New Bottom Plate_v3 (Autodesk Fusion 360 design; units mm, degrees)
Autodesk Fusion 360 part; units mm, degrees
note: some values were not read from the file. Set by a fixed rule: which sketch regions a step uses.
sketch "Reference" plane through (0, 0, 0) normal (0, 0, 1) x (1, 0, 0)
  line L0 (298.2751, -95.25) -> (298.2751, -113.3)
  line L1 (298.275, 1) -> (298.275, -57.15)
  line L2 (298.275, -57.15) -> (298.275, -57.15)
  line L3 (304.5217, -115.3) -> (303.775, 3)
  line L4 (179.47, 0) -> (290.235, 0)
  line L5 (290.2351, -112.3) -> (230.642, -112.3)
  line L6 (290.235, 1) -> (298.275, 1)
  line L7 (290.235, 0) -> (298.275, 0)
  line L8 (290.2351, -112.3) -> (298.2751, -112.3)
  arc A0 (302.0217, -117.8) -> (304.5217, -115.3) centre (302.0374, -115.3157) ccw
  line L9 (298.2751, -57.15) -> (298.2751, -74.2)
  line L10 (171.43, 0) -> (171.43, 1)
  line L11 (230.642, -112.3) -> (230.642, -113.3)
  line L12 (222.602, -113.3) -> (222.602, -112.3)
  arc A1 (303.775, 3) -> (301.275, 5.5) centre (301.275, 3) ccw
  line L13 (-28.337, -112.3) -> (-29.3375, -112.3)
  line L14 (-28.3375, 1.5) -> (-28.3375, 3)
  line L15 (-28.337, 1.5) -> (-6.3413, 1.5)
  line L16 (230.642, -112.3) -> (230.642, -113.3)
  line L17 (230.642, -113.3) -> (222.602, -113.3)
  line L18 (-36.12, -117.7958) -> (-31.338, -117.8)
  line L19 (222.602, -113.3) -> (222.602, -112.3)
  line L20 (-28.337, -113.3) -> (-28.337, -112.3)
  line L21 (-29.3375, -113.3) -> (-29.338, -113.3)
  arc A2 (-38.6178, -115.2937) -> (-36.12, -117.7958) centre (-36.1178, -115.2958) ccw
  line L22 (57.336, -112.3) -> (-20.297, -112.3)
  line L23 (8.02, 1) -> (8.02, 0)
  line L24 (-29.3375, -112.3) -> (-29.3375, -113.3)
  line L25 (-33.0995, -112.3) -> (-33.0995, 1.5)
  line L26 (-29.338, -112.3) -> (-33.0995, -112.3)
  line L27 (57.336, -113.3) -> (57.336, -112.3)
  line L28 (-20.297, -113.3) -> (-28.337, -113.3)
  line L29 (-29.338, -113.3) -> (-29.338, -112.3)
  line L30 (-20.297, -112.3) -> (-20.297, -113.3)
  line L31 (301.275, 5.5) -> (-36.0995, 5.5)
  line L32 (-38.5995, -94.25) -> (-38.6178, -115.2937)
  line L33 (298.2751, -76.2) -> (298.2751, -93.25)
  line L34 (298.275, -95.25) -> (298.275, -95.25)
  line L35 (298.275, -76.2) -> (298.275, -76.2)
  line L36 (-6.3413, 1.5) -> (-6.3413, 0)
  line L37 (-38.5995, 3) -> (-38.5995, -94.25)
  arc A3 (303.775, 3) -> (301.275, 5.5) centre (301.275, 3) ccw
  line L38 (298.2751, -74.2) -> (298.275, -74.2)
  line L39 (-28.337, 3) -> (-28.337, 1.5)
  line L40 (-33.0995, 1.5) -> (-28.3375, 1.5)
  line L41 (-0.02, 0) -> (-0.02, 1)
  arc A4 (-36.0995, 5.5) -> (-38.5995, 3) centre (-36.0995, 3) ccw
  line L42 (-31.338, -117.8) -> (302.0217, -117.8)
  line L43 (-6.3413, 0) -> (-0.02, 0)
  line L44 (298.275, -57.15) -> (298.275, -57.15)
  line L45 (-0.02, 1) -> (8.02, 1)
  line L46 (8.02, 0) -> (171.43, 0)
  line L47 (-28.3375, 3) -> (-28.337, 3)
  line L48 (290.235, 0) -> (290.235, 1)
  line L49 (290.235, 1) -> (298.275, 1)
  line L50 (298.2751, -57.15) -> (298.2751, -74.2)
  line L51 (298.275, 1) -> (298.275, -57.15)
  line L52 (222.602, -112.3) -> (65.376, -112.3)
  line L53 (-33.0995, -112.3) -> (-33.0995, 1.5)
  line L54 (301.275, 5.5) -> (-36.0995, 5.5)
  line L55 (-31.338, -117.8) -> (302.0217, -117.8)
  line L56 (57.336, -112.3) -> (-20.297, -112.3)
  line L57 (8.02, 0) -> (171.43, 0)
  line L58 (290.2351, -112.3) -> (230.642, -112.3)
  line L59 (298.2751, -95.25) -> (298.2751, -113.3)
  line L60 (298.275, -76.2) -> (298.275, -76.2)
  line L61 (298.275, -74.2) -> (298.275, -76.2)
  line L62 (298.2751, -76.2) -> (298.2751, -93.25)
  line L63 (298.2751, -93.25) -> (298.275, -93.25)
  line L64 (298.275, -93.25) -> (298.275, -95.25)
  line L65 (290.2351, -113.3) -> (290.2351, -112.3)
  arc A5 (302.0217, -117.8) -> (304.5217, -115.3) centre (302.0374, -115.3157) ccw
  line L66 (179.47, 0) -> (290.235, 0)
  line L67 (298.2751, -113.3) -> (290.2351, -113.3)
  line L68 (304.5217, -115.3) -> (303.775, 3)
  line L69 (298.275, -95.25) -> (298.275, -95.25)
  line L70 (57.336, -113.3) -> (57.336, -112.3)
  line L71 (65.376, -113.3) -> (57.336, -113.3)
  line L72 (-29.338, -113.3) -> (-29.338, -112.3)
  line L73 (-6.3413, 1.5) -> (-6.3413, 0)
  line L74 (-29.3375, -113.3) -> (-29.338, -113.3)
  line L75 (-29.3375, -112.3) -> (-29.3375, -113.3)
  line L76 (-28.3375, 1.5) -> (-28.3375, 3)
  line L77 (-28.337, 1.5) -> (-6.3413, 1.5)
  line L78 (-28.337, -112.3) -> (-29.3375, -112.3)
  line L79 (-28.337, -113.3) -> (-28.337, -112.3)
  line L80 (-28.3375, 3) -> (-28.337, 3)
  line L81 (-20.297, -113.3) -> (-28.337, -113.3)
  line L82 (65.376, -112.3) -> (65.376, -113.3)
  line L83 (-20.297, -112.3) -> (-20.297, -113.3)
  line L84 (-29.338, -112.3) -> (-33.0995, -112.3)
  line L85 (8.02, 1) -> (8.02, 0)
  line L86 (-28.337, 3) -> (-28.337, 1.5)
  arc A6 (-38.6178, -115.2937) -> (-36.12, -117.7958) centre (-36.1178, -115.2958) ccw
  line L87 (-38.5995, -94.25) -> (-38.6178, -115.2937)
  line L88 (-38.5995, 3) -> (-38.5995, -94.25)
  line L89 (-0.02, 0) -> (-0.02, 1)
  line L90 (-33.0995, 1.5) -> (-28.3375, 1.5)
  line L91 (-6.3413, 0) -> (-0.02, 0)
  arc A7 (-36.0995, 5.5) -> (-38.5995, 3) centre (-36.0995, 3) ccw
  line L92 (-0.02, 1) -> (8.02, 1)
  line L93 (-36.12, -117.7958) -> (-31.338, -117.8)
  line L94 (298.275, -93.25) -> (298.275, -95.25)
  line L95 (298.2751, -113.3) -> (290.2351, -113.3)
  line L96 (290.2351, -113.3) -> (290.2351, -112.3)
  line L97 (298.2751, -93.25) -> (298.275, -93.25)
  line L98 (298.275, -74.2) -> (298.275, -76.2)
  line L99 (298.2751, -74.2) -> (298.275, -74.2)
  line L100 (290.235, 0) -> (290.235, 1)
  line L101 (179.47, 1) -> (179.47, 0)
  line L102 (230.642, -113.3) -> (222.602, -113.3)
  line L103 (179.47, 1) -> (179.47, 0)
  line L104 (171.43, 1) -> (179.47, 1)
  line L105 (222.602, -112.3) -> (65.376, -112.3)
  line L106 (65.376, -112.3) -> (65.376, -113.3)
  line L107 (65.376, -113.3) -> (57.336, -113.3)
  line L108 (171.43, 0) -> (171.43, 1)
  line L109 (171.43, 1) -> (179.47, 1)
  dimension "d29" = 5.5
  dimension "d30" = 5.5
  dimension "d31" = 6.2339
  dimension "d32" = 5.5125
  dimension "d33" = 5.5
  dimension "d34" = 6.2276
  dimension "d35" = 5.5188
  constraint coincident L5.start L8.start
  constraint perpendicular L0 L8
  constraint coincident L8.end L59
  constraint coincident L4.end L7.start
  constraint perpendicular L7 L48
  constraint coincident L7.end L51
  measures "d29" distance of L42 L58
  measures "d30" distance of L4 L31
  measures "d31" distance of L0.end L3
  measures "d32" distance of L1.start L3
  measures "d33" distance of L25 L37
  measures "d34" distance of L8.end L3
  measures "d35" distance of L7.end L68
sketch "FlatPlateSketch" plane through (0, 0, 0) normal (0, 0, 1) x (1, 0, 0)
  line L0 (298.2751, -95.25) -> (298.2751, -113.3)
  line L1 (298.275, 1) -> (298.275, -57.15)
  line L2 (298.275, -57.15) -> (298.275, -57.15)
  line L3 (304.5217, -115.3) -> (303.775, 3)
  line L4 (179.47, 0) -> (290.235, 0)
  line L5 (290.2351, -112.3) -> (230.642, -112.3)
  line L6 (290.235, 1) -> (298.275, 1)
  line L7 (290.235, 0) -> (298.275, 0)
  line L8 (290.2351, -112.3) -> (298.2751, -112.3)
  arc A0 (302.0217, -117.8) -> (304.5217, -115.3) centre (302.0374, -115.3157) ccw
  line L9 (298.2751, -57.15) -> (298.2751, -74.2)
  line L10 (171.43, 0) -> (171.43, 1)
  line L11 (230.642, -112.3) -> (230.642, -113.3)
  line L12 (222.602, -113.3) -> (222.602, -112.3)
  arc A1 (303.775, 3) -> (301.275, 5.5) centre (301.275, 3) ccw
  line L13 (-28.337, -112.3) -> (-29.3375, -112.3)
  line L14 (-28.3375, 1.5) -> (-28.3375, 3)
  line L15 (-28.337, 1.5) -> (-6.3413, 1.5)
  line L16 (230.642, -112.3) -> (230.642, -113.3)
  line L17 (230.642, -113.3) -> (222.602, -113.3)
  line L18 (-36.12, -117.7958) -> (-31.338, -117.8)
  line L19 (222.602, -113.3) -> (222.602, -112.3)
  line L20 (-28.337, -113.3) -> (-28.337, -112.3)
  line L21 (-29.3375, -113.3) -> (-29.338, -113.3)
  arc A2 (-38.6178, -115.2937) -> (-36.12, -117.7958) centre (-36.1178, -115.2958) ccw
  line L22 (57.336, -112.3) -> (-20.297, -112.3)
  line L23 (8.02, 1) -> (8.02, 0)
  line L24 (-29.3375, -112.3) -> (-29.3375, -113.3)
  line L25 (-33.0995, -112.3) -> (-33.0995, 1.5)
  line L26 (-29.338, -112.3) -> (-33.0995, -112.3)
  line L27 (57.336, -113.3) -> (57.336, -112.3)
  line L28 (-20.297, -113.3) -> (-28.337, -113.3)
  line L29 (-29.338, -113.3) -> (-29.338, -112.3)
  line L30 (-20.297, -112.3) -> (-20.297, -113.3)
  line L31 (301.275, 5.5) -> (-36.0995, 5.5)
  line L32 (-38.5995, -94.25) -> (-38.6178, -115.2937)
  line L33 (298.2751, -76.2) -> (298.2751, -93.25)
  line L34 (298.275, -95.25) -> (298.275, -95.25)
  line L35 (298.275, -76.2) -> (298.275, -76.2)
  line L36 (-6.3413, 1.5) -> (-6.3413, 0)
  line L37 (-38.5995, 3) -> (-38.5995, -94.25)
  arc A3 (303.775, 3) -> (301.275, 5.5) centre (301.275, 3) ccw
  line L38 (298.2751, -74.2) -> (298.275, -74.2)
  line L39 (-28.337, 3) -> (-28.337, 1.5)
  line L40 (-33.0995, 1.5) -> (-28.3375, 1.5)
  line L41 (-0.02, 0) -> (-0.02, 1)
  arc A4 (-36.0995, 5.5) -> (-38.5995, 3) centre (-36.0995, 3) ccw
  line L42 (-31.338, -117.8) -> (302.0217, -117.8)
  line L43 (-6.3413, 0) -> (-0.02, 0)
  line L44 (298.275, -57.15) -> (298.275, -57.15)
  line L45 (-0.02, 1) -> (8.02, 1)
  line L46 (8.02, 0) -> (171.43, 0)
  line L47 (-28.3375, 3) -> (-28.337, 3)
  line L48 (290.235, 0) -> (290.235, 1)
  line L49 (290.235, 1) -> (298.275, 1)
  line L50 (298.2751, -57.15) -> (298.2751, -74.2)
  line L51 (298.275, 1) -> (298.275, -57.15)
  line L52 (222.602, -112.3) -> (65.376, -112.3)
  line L53 (-33.0995, -112.3) -> (-33.0995, 1.5)
  line L54 (301.275, 5.5) -> (-36.0995, 5.5)
  line L55 (-31.338, -117.8) -> (302.0217, -117.8)
  line L56 (57.336, -112.3) -> (-20.297, -112.3)
  line L57 (8.02, 0) -> (171.43, 0)
  line L58 (290.2351, -112.3) -> (230.642, -112.3)
  line L59 (298.2751, -95.25) -> (298.2751, -113.3)
  line L60 (298.275, -76.2) -> (298.275, -76.2)
  line L61 (298.275, -74.2) -> (298.275, -76.2)
  line L62 (298.2751, -76.2) -> (298.2751, -93.25)
  line L63 (298.2751, -93.25) -> (298.275, -93.25)
  line L64 (298.275, -93.25) -> (298.275, -95.25)
  line L65 (290.2351, -113.3) -> (290.2351, -112.3)
  arc A5 (302.0217, -117.8) -> (304.5217, -115.3) centre (302.0374, -115.3157) ccw
  line L66 (179.47, 0) -> (290.235, 0)
  line L67 (298.2751, -113.3) -> (290.2351, -113.3)
  line L68 (304.5217, -115.3) -> (303.775, 3)
  line L69 (298.275, -95.25) -> (298.275, -95.25)
  line L70 (57.336, -113.3) -> (57.336, -112.3)
  line L71 (65.376, -113.3) -> (57.336, -113.3)
  line L72 (-29.338, -113.3) -> (-29.338, -112.3)
  line L73 (-6.3413, 1.5) -> (-6.3413, 0)
  line L74 (-29.3375, -113.3) -> (-29.338, -113.3)
  line L75 (-29.3375, -112.3) -> (-29.3375, -113.3)
  line L76 (-28.3375, 1.5) -> (-28.3375, 3)
  line L77 (-28.337, 1.5) -> (-6.3413, 1.5)
  line L78 (-28.337, -112.3) -> (-29.3375, -112.3)
  line L79 (-28.337, -113.3) -> (-28.337, -112.3)
  line L80 (-28.3375, 3) -> (-28.337, 3)
  line L81 (-20.297, -113.3) -> (-28.337, -113.3)
  line L82 (65.376, -112.3) -> (65.376, -113.3)
  line L83 (-20.297, -112.3) -> (-20.297, -113.3)
  line L84 (-29.338, -112.3) -> (-33.0995, -112.3)
  line L85 (8.02, 1) -> (8.02, 0)
  line L86 (-28.337, 3) -> (-28.337, 1.5)
  arc A6 (-38.6178, -115.2937) -> (-36.12, -117.7958) centre (-36.1178, -115.2958) ccw
  line L87 (-38.5995, -94.25) -> (-38.6178, -115.2937)
  line L88 (-38.5995, 3) -> (-38.5995, -94.25)
  line L89 (-0.02, 0) -> (-0.02, 1)
  line L90 (-33.0995, 1.5) -> (-28.3375, 1.5)
  line L91 (-6.3413, 0) -> (-0.02, 0)
  arc A7 (-36.0995, 5.5) -> (-38.5995, 3) centre (-36.0995, 3) ccw
  line L92 (-0.02, 1) -> (8.02, 1)
  line L93 (-36.12, -117.7958) -> (-31.338, -117.8)
  line L94 (298.275, -93.25) -> (298.275, -95.25)
  line L95 (298.2751, -113.3) -> (290.2351, -113.3)
  line L96 (290.2351, -113.3) -> (290.2351, -112.3)
  line L97 (298.2751, -93.25) -> (298.275, -93.25)
  line L98 (298.275, -74.2) -> (298.275, -76.2)
  line L99 (298.2751, -74.2) -> (298.275, -74.2)
  line L100 (290.235, 0) -> (290.235, 1)
  line L101 (179.47, 1) -> (179.47, 0)
  line L102 (230.642, -113.3) -> (222.602, -113.3)
  line L103 (179.47, 1) -> (179.47, 0)
  line L104 (171.43, 1) -> (179.47, 1)
  line L105 (222.602, -112.3) -> (65.376, -112.3)
  line L106 (65.376, -112.3) -> (65.376, -113.3)
  line L107 (65.376, -113.3) -> (57.336, -113.3)
  line L108 (171.43, 0) -> (171.43, 1)
  line L109 (171.43, 1) -> (179.47, 1)
  dimension "d36" = 5.5
  dimension "d37" = 5.5
  dimension "d38" = 6.2339
  dimension "d39" = 5.5125
  dimension "d40" = 5.5
  dimension "d41" = 6.2276
  dimension "d42" = 5.5188
  constraint coincident L5.start L8.start
  constraint perpendicular L0 L8
  constraint coincident L8.end L59
  constraint coincident L4.end L7.start
  constraint perpendicular L7 L48
  constraint coincident L7.end L51
  measures "d36" distance of L42 L58
  measures "d37" distance of L4 L31
  measures "d38" distance of L0.end L3
  measures "d39" distance of L1.start L3
  measures "d40" distance of L25 L37
  measures "d41" distance of L8.end L3
  measures "d42" distance of L7.end L68
sketch "Sketch7" plane through (0, 0, 0) normal (0, 0, 1) x (1, 0, 0)
  line L0 (298.2751, -95.25) -> (298.2751, -113.3)
  line L1 (298.275, 1) -> (298.275, -57.15)
  line L2 (298.275, -57.15) -> (298.275, -57.15)
  line L3 (304.5217, -115.3) -> (303.775, 3)
  line L4 (179.47, 0) -> (290.235, 0)
  line L5 (290.2351, -112.3) -> (230.642, -112.3)
  line L6 (290.235, 1) -> (298.275, 1)
  line L7 (290.235, 0) -> (298.275, 0)
  line L8 (290.2351, -112.3) -> (298.2751, -112.3)
  arc A0 (302.0217, -117.8) -> (304.5217, -115.3) centre (302.0374, -115.3157) ccw
  line L9 (298.2751, -57.15) -> (298.2751, -74.2)
  line L10 (171.43, 0) -> (171.43, 1)
  line L11 (230.642, -112.3) -> (230.642, -113.3)
  line L12 (222.602, -113.3) -> (222.602, -112.3)
  arc A1 (303.775, 3) -> (301.275, 5.5) centre (301.275, 3) ccw
  line L13 (-28.337, -112.3) -> (-29.3375, -112.3)
  line L14 (-28.3375, 1.5) -> (-28.3375, 3)
  line L15 (-28.337, 1.5) -> (-6.3413, 1.5)
  line L16 (230.642, -112.3) -> (230.642, -113.3)
  line L17 (230.642, -113.3) -> (222.602, -113.3)
  line L18 (-36.12, -117.7958) -> (-31.338, -117.8)
  line L19 (222.602, -113.3) -> (222.602, -112.3)
  line L20 (-28.337, -113.3) -> (-28.337, -112.3)
  line L21 (-29.3375, -113.3) -> (-29.338, -113.3)
  arc A2 (-38.6178, -115.2937) -> (-36.12, -117.7958) centre (-36.1178, -115.2958) ccw
  line L22 (57.336, -112.3) -> (-20.297, -112.3)
  line L23 (8.02, 1) -> (8.02, 0)
  line L24 (-29.3375, -112.3) -> (-29.3375, -113.3)
  line L25 (-33.0995, -112.3) -> (-33.0995, 1.5)
  line L26 (-29.338, -112.3) -> (-33.0995, -112.3)
  line L27 (57.336, -113.3) -> (57.336, -112.3)
  line L28 (-20.297, -113.3) -> (-28.337, -113.3)
  line L29 (-29.338, -113.3) -> (-29.338, -112.3)
  line L30 (-20.297, -112.3) -> (-20.297, -113.3)
  line L31 (301.275, 5.5) -> (-36.0995, 5.5)
  line L32 (-38.5995, -94.25) -> (-38.6178, -115.2937)
  line L33 (298.2751, -76.2) -> (298.2751, -93.25)
  line L34 (298.275, -95.25) -> (298.275, -95.25)
  line L35 (298.275, -76.2) -> (298.275, -76.2)
  line L36 (-6.3413, 1.5) -> (-6.3413, 0)
  line L37 (-38.5995, 3) -> (-38.5995, -94.25)
  arc A3 (303.775, 3) -> (301.275, 5.5) centre (301.275, 3) ccw
  line L38 (298.2751, -74.2) -> (298.275, -74.2)
  line L39 (-28.337, 3) -> (-28.337, 1.5)
  line L40 (-33.0995, 1.5) -> (-28.3375, 1.5)
  line L41 (-0.02, 0) -> (-0.02, 1)
  arc A4 (-36.0995, 5.5) -> (-38.5995, 3) centre (-36.0995, 3) ccw
  line L42 (-31.338, -117.8) -> (302.0217, -117.8)
  line L43 (-6.3413, 0) -> (-0.02, 0)
  line L44 (298.275, -57.15) -> (298.275, -57.15)
  line L45 (-0.02, 1) -> (8.02, 1)
  line L46 (8.02, 0) -> (171.43, 0)
  line L47 (-28.3375, 3) -> (-28.337, 3)
  line L48 (290.235, 0) -> (290.235, 1)
  line L49 (290.235, 1) -> (298.275, 1)
  line L50 (298.2751, -57.15) -> (298.2751, -74.2)
  line L51 (298.275, 1) -> (298.275, -57.15)
  line L52 (222.602, -112.3) -> (65.376, -112.3)
  line L53 (-33.0995, -112.3) -> (-33.0995, 1.5)
  line L54 (301.275, 5.5) -> (-36.0995, 5.5)
  line L55 (-31.338, -117.8) -> (302.0217, -117.8)
  line L56 (57.336, -112.3) -> (-20.297, -112.3)
  line L57 (8.02, 0) -> (171.43, 0)
  line L58 (290.2351, -112.3) -> (230.642, -112.3)
  line L59 (298.2751, -95.25) -> (298.2751, -113.3)
  line L60 (298.275, -76.2) -> (298.275, -76.2)
  line L61 (298.275, -74.2) -> (298.275, -76.2)
  line L62 (298.2751, -76.2) -> (298.2751, -93.25)
  line L63 (298.2751, -93.25) -> (298.275, -93.25)
  line L64 (298.275, -93.25) -> (298.275, -95.25)
  line L65 (290.2351, -113.3) -> (290.2351, -112.3)
  arc A5 (302.0217, -117.8) -> (304.5217, -115.3) centre (302.0374, -115.3157) ccw
  line L66 (179.47, 0) -> (290.235, 0)
  line L67 (298.2751, -113.3) -> (290.2351, -113.3)
  line L68 (304.5217, -115.3) -> (303.775, 3)
  line L69 (298.275, -95.25) -> (298.275, -95.25)
  line L70 (57.336, -113.3) -> (57.336, -112.3)
  line L71 (65.376, -113.3) -> (57.336, -113.3)
  line L72 (-29.338, -113.3) -> (-29.338, -112.3)
  line L73 (-6.3413, 1.5) -> (-6.3413, 0)
  line L74 (-29.3375, -113.3) -> (-29.338, -113.3)
  line L75 (-29.3375, -112.3) -> (-29.3375, -113.3)
  line L76 (-28.3375, 1.5) -> (-28.3375, 3)
  line L77 (-28.337, 1.5) -> (-6.3413, 1.5)
  line L78 (-28.337, -112.3) -> (-29.3375, -112.3)
  line L79 (-28.337, -113.3) -> (-28.337, -112.3)
  line L80 (-28.3375, 3) -> (-28.337, 3)
  line L81 (-20.297, -113.3) -> (-28.337, -113.3)
  line L82 (65.376, -112.3) -> (65.376, -113.3)
  line L83 (-20.297, -112.3) -> (-20.297, -113.3)
  line L84 (-29.338, -112.3) -> (-33.0995, -112.3)
  line L85 (8.02, 1) -> (8.02, 0)
  line L86 (-28.337, 3) -> (-28.337, 1.5)
  arc A6 (-38.6178, -115.2937) -> (-36.12, -117.7958) centre (-36.1178, -115.2958) ccw
  line L87 (-38.5995, -94.25) -> (-38.6178, -115.2937)
  line L88 (-38.5995, 3) -> (-38.5995, -94.25)
  line L89 (-0.02, 0) -> (-0.02, 1)
  line L90 (-33.0995, 1.5) -> (-28.3375, 1.5)
  line L91 (-6.3413, 0) -> (-0.02, 0)
  arc A7 (-36.0995, 5.5) -> (-38.5995, 3) centre (-36.0995, 3) ccw
  line L92 (-0.02, 1) -> (8.02, 1)
  line L93 (-36.12, -117.7958) -> (-31.338, -117.8)
  line L94 (298.275, -93.25) -> (298.275, -95.25)
  line L95 (298.2751, -113.3) -> (290.2351, -113.3)
  line L96 (290.2351, -113.3) -> (290.2351, -112.3)
  line L97 (298.2751, -93.25) -> (298.275, -93.25)
  line L98 (298.275, -74.2) -> (298.275, -76.2)
  line L99 (298.2751, -74.2) -> (298.275, -74.2)
  line L100 (290.235, 0) -> (290.235, 1)
  line L101 (179.47, 1) -> (179.47, 0)
  line L102 (230.642, -113.3) -> (222.602, -113.3)
  line L103 (179.47, 1) -> (179.47, 0)
  line L104 (171.43, 1) -> (179.47, 1)
  line L105 (222.602, -112.3) -> (65.376, -112.3)
  line L106 (65.376, -112.3) -> (65.376, -113.3)
  line L107 (65.376, -113.3) -> (57.336, -113.3)
  line L108 (171.43, 0) -> (171.43, 1)
  line L109 (171.43, 1) -> (179.47, 1)
  dimension "d45" = 5.5
  dimension "d46" = 5.5
  dimension "d47" = 6.2339
  dimension "d48" = 5.5125
  dimension "d49" = 5.5
  dimension "d50" = 6.2276
  dimension "d51" = 5.5188
  constraint coincident L5.start L8.start
  constraint perpendicular L0 L8
  constraint coincident L8.end L59
  constraint coincident L4.end L7.start
  constraint perpendicular L7 L48
  constraint coincident L7.end L51
  measures "d45" distance of L42 L58
  measures "d46" distance of L4 L31
  measures "d47" distance of L0.end L3
  measures "d48" distance of L1.start L3
  measures "d49" distance of L25 L37
  measures "d50" distance of L8.end L3
  measures "d51" distance of L7.end L68
extrude "Extrude4" add sketch "FlatPlateSketch" against normal blind 1 contours L0 L1 L4 L5 L7 L8 L9 L10 L11 L12 L13 L15 L16 L17 L19 L20 L22 L23 L25 L26 L27 L28 L30 L33 L36 L40 L41 L43 L45 L46 L50 L51 L52 L53 L56 L57 L58 L59 L61 L62 L64 L66 L70 L71 L73 L77 L78 L79 L81 L82 L83 L84 L85 L89 L90 L91 L92 L94 L98 L101 L102 L103 L104 L105 L106 L107 L108 L109 | L0 L8 L59 L65 L67 L95 L96 | L1 L6 L7 L48 L49 L51 L100 | L3 A0 A1 L18 A2 L31 L32 L37 A3 A4 L42 L54 L55 A5 L68 A6 L87 L88 A7 L93
sketch "Sketch8" plane through (0, 0, 0) normal (0, 0, 1) x (1, 0, 0)
  line L0 (298.2751, -95.25) -> (298.2751, -113.3)
  line L1 (298.275, 1) -> (298.275, -57.15)
  line L2 (298.275, -57.15) -> (298.275, -57.15)
  line L3 (304.5217, -115.3) -> (303.775, 3)
  line L4 (179.47, 0) -> (290.235, 0)
  line L5 (290.2351, -112.3) -> (230.642, -112.3)
  line L6 (290.235, 1) -> (298.275, 1)
  line L7 (290.235, 0) -> (298.275, 0)
  line L8 (290.2351, -112.3) -> (298.2751, -112.3)
  arc A0 (302.0217, -117.8) -> (304.5217, -115.3) centre (302.0374, -115.3157) ccw
  line L9 (298.2751, -57.15) -> (298.2751, -74.2)
  line L10 (171.43, 0) -> (171.43, 1)
  line L11 (230.642, -112.3) -> (230.642, -113.3)
  line L12 (222.602, -113.3) -> (222.602, -112.3)
  arc A1 (303.775, 3) -> (301.275, 5.5) centre (301.275, 3) ccw
  line L13 (-28.337, -112.3) -> (-29.3375, -112.3)
  line L14 (-28.3375, 1.5) -> (-28.3375, 3)
  line L15 (-28.337, 1.5) -> (-6.3413, 1.5)
  line L16 (230.642, -112.3) -> (230.642, -113.3)
  line L17 (230.642, -113.3) -> (222.602, -113.3)
  line L18 (-36.12, -117.7958) -> (-31.338, -117.8)
  line L19 (222.602, -113.3) -> (222.602, -112.3)
  line L20 (-28.337, -113.3) -> (-28.337, -112.3)
  line L21 (-29.3375, -113.3) -> (-29.338, -113.3)
  arc A2 (-38.6178, -115.2937) -> (-36.12, -117.7958) centre (-36.1178, -115.2958) ccw
  line L22 (57.336, -112.3) -> (-20.297, -112.3)
  line L23 (8.02, 1) -> (8.02, 0)
  line L24 (-29.3375, -112.3) -> (-29.3375, -113.3)
  line L25 (-33.0995, -112.3) -> (-33.0995, 1.5)
  line L26 (-29.338, -112.3) -> (-33.0995, -112.3)
  line L27 (57.336, -113.3) -> (57.336, -112.3)
  line L28 (-20.297, -113.3) -> (-28.337, -113.3)
  line L29 (-29.338, -113.3) -> (-29.338, -112.3)
  line L30 (-20.297, -112.3) -> (-20.297, -113.3)
  line L31 (301.275, 5.5) -> (-36.0995, 5.5)
  line L32 (-38.5995, -94.25) -> (-38.6178, -115.2937)
  line L33 (298.2751, -76.2) -> (298.2751, -93.25)
  line L34 (298.275, -95.25) -> (298.275, -95.25)
  line L35 (298.275, -76.2) -> (298.275, -76.2)
  line L36 (-6.3413, 1.5) -> (-6.3413, 0)
  line L37 (-38.5995, 3) -> (-38.5995, -94.25)
  arc A3 (303.775, 3) -> (301.275, 5.5) centre (301.275, 3) ccw
  line L38 (298.2751, -74.2) -> (298.275, -74.2)
  line L39 (-28.337, 3) -> (-28.337, 1.5)
  line L40 (-33.0995, 1.5) -> (-28.3375, 1.5)
  line L41 (-0.02, 0) -> (-0.02, 1)
  arc A4 (-36.0995, 5.5) -> (-38.5995, 3) centre (-36.0995, 3) ccw
  line L42 (-31.338, -117.8) -> (302.0217, -117.8)
  line L43 (-6.3413, 0) -> (-0.02, 0)
  line L44 (298.275, -57.15) -> (298.275, -57.15)
  line L45 (-0.02, 1) -> (8.02, 1)
  line L46 (8.02, 0) -> (171.43, 0)
  line L47 (-28.3375, 3) -> (-28.337, 3)
  line L48 (290.235, 0) -> (290.235, 1)
  line L49 (290.235, 1) -> (298.275, 1)
  line L50 (298.2751, -57.15) -> (298.2751, -74.2)
  line L51 (298.275, 1) -> (298.275, -57.15)
  line L52 (222.602, -112.3) -> (65.376, -112.3)
  line L53 (-33.0995, -112.3) -> (-33.0995, 1.5)
  line L54 (301.275, 5.5) -> (-36.0995, 5.5)
  line L55 (-31.338, -117.8) -> (302.0217, -117.8)
  line L56 (57.336, -112.3) -> (-20.297, -112.3)
  line L57 (8.02, 0) -> (171.43, 0)
  line L58 (290.2351, -112.3) -> (230.642, -112.3)
  line L59 (298.2751, -95.25) -> (298.2751, -113.3)
  line L60 (298.275, -76.2) -> (298.275, -76.2)
  line L61 (298.275, -74.2) -> (298.275, -76.2)
  line L62 (298.2751, -76.2) -> (298.2751, -93.25)
  line L63 (298.2751, -93.25) -> (298.275, -93.25)
  line L64 (298.275, -93.25) -> (298.275, -95.25)
  line L65 (290.2351, -113.3) -> (290.2351, -112.3)
  arc A5 (302.0217, -117.8) -> (304.5217, -115.3) centre (302.0374, -115.3157) ccw
  line L66 (179.47, 0) -> (290.235, 0)
  line L67 (298.2751, -113.3) -> (290.2351, -113.3)
  line L68 (304.5217, -115.3) -> (303.775, 3)
  line L69 (298.275, -95.25) -> (298.275, -95.25)
  line L70 (57.336, -113.3) -> (57.336, -112.3)
  line L71 (65.376, -113.3) -> (57.336, -113.3)
  line L72 (-29.338, -113.3) -> (-29.338, -112.3)
  line L73 (-6.3413, 1.5) -> (-6.3413, 0)
  line L74 (-29.3375, -113.3) -> (-29.338, -113.3)
  line L75 (-29.3375, -112.3) -> (-29.3375, -113.3)
  line L76 (-28.3375, 1.5) -> (-28.3375, 3)
  line L77 (-28.337, 1.5) -> (-6.3413, 1.5)
  line L78 (-28.337, -112.3) -> (-29.3375, -112.3)
  line L79 (-28.337, -113.3) -> (-28.337, -112.3)
  line L80 (-28.3375, 3) -> (-28.337, 3)
  line L81 (-20.297, -113.3) -> (-28.337, -113.3)
  line L82 (65.376, -112.3) -> (65.376, -113.3)
  line L83 (-20.297, -112.3) -> (-20.297, -113.3)
  line L84 (-29.338, -112.3) -> (-33.0995, -112.3)
  line L85 (8.02, 1) -> (8.02, 0)
  line L86 (-28.337, 3) -> (-28.337, 1.5)
  arc A6 (-38.6178, -115.2937) -> (-36.12, -117.7958) centre (-36.1178, -115.2958) ccw
  line L87 (-38.5995, -94.25) -> (-38.6178, -115.2937)
  line L88 (-38.5995, 3) -> (-38.5995, -94.25)
  line L89 (-0.02, 0) -> (-0.02, 1)
  line L90 (-33.0995, 1.5) -> (-28.3375, 1.5)
  line L91 (-6.3413, 0) -> (-0.02, 0)
  arc A7 (-36.0995, 5.5) -> (-38.5995, 3) centre (-36.0995, 3) ccw
  line L92 (-0.02, 1) -> (8.02, 1)
  line L93 (-36.12, -117.7958) -> (-31.338, -117.8)
  line L94 (298.275, -93.25) -> (298.275, -95.25)
  line L95 (298.2751, -113.3) -> (290.2351, -113.3)
  line L96 (290.2351, -113.3) -> (290.2351, -112.3)
  line L97 (298.2751, -93.25) -> (298.275, -93.25)
  line L98 (298.275, -74.2) -> (298.275, -76.2)
  line L99 (298.2751, -74.2) -> (298.275, -74.2)
  line L100 (290.235, 0) -> (290.235, 1)
  line L101 (179.47, 1) -> (179.47, 0)
  line L102 (230.642, -113.3) -> (222.602, -113.3)
  line L103 (179.47, 1) -> (179.47, 0)
  line L104 (171.43, 1) -> (179.47, 1)
  line L105 (222.602, -112.3) -> (65.376, -112.3)
  line L106 (65.376, -112.3) -> (65.376, -113.3)
  line L107 (65.376, -113.3) -> (57.336, -113.3)
  line L108 (171.43, 0) -> (171.43, 1)
  line L109 (171.43, 1) -> (179.47, 1)
  dimension "d54" = 5.5
  dimension "d55" = 5.5
  dimension "d56" = 6.2339
  dimension "d57" = 5.5125
  dimension "d58" = 5.5
  dimension "d59" = 6.2276
  dimension "d60" = 5.5188
  constraint coincident L5.start L8.start
  constraint perpendicular L0 L8
  constraint coincident L8.end L59
  constraint coincident L4.end L7.start
  constraint perpendicular L7 L48
  constraint coincident L7.end L51
  measures "d54" distance of L42 L58
  measures "d55" distance of L4 L31
  measures "d56" distance of L0.end L3
  measures "d57" distance of L1.start L3
  measures "d58" distance of L25 L37
  measures "d59" distance of L8.end L3
  measures "d60" distance of L7.end L68
sketch "Sketch9" plane through (0, 0, 0) normal (0, 0, 1) x (1, 0, 0)
  line L0 (298.2751, -95.25) -> (298.2751, -113.3)
  line L1 (298.275, 1) -> (298.275, -57.15)
  line L2 (298.275, -57.15) -> (298.275, -57.15)
  line L3 (304.5217, -115.3) -> (303.775, 3)
  line L4 (179.47, 0) -> (290.235, 0)
  line L5 (290.2351, -112.3) -> (230.642, -112.3)
  line L6 (290.235, 1) -> (298.275, 1)
  line L7 (290.235, 0) -> (298.275, 0)
  line L8 (290.2351, -112.3) -> (298.2751, -112.3)
  arc A0 (302.0217, -117.8) -> (304.5217, -115.3) centre (302.0374, -115.3157) ccw
  line L9 (298.2751, -57.15) -> (298.2751, -74.2)
  line L10 (171.43, 0) -> (171.43, 1)
  line L11 (230.642, -112.3) -> (230.642, -113.3)
  line L12 (222.602, -113.3) -> (222.602, -112.3)
  arc A1 (303.775, 3) -> (301.275, 5.5) centre (301.275, 3) ccw
  line L13 (-28.337, -112.3) -> (-29.3375, -112.3)
  line L14 (-28.3375, 1.5) -> (-28.3375, 3)
  line L15 (-28.337, 1.5) -> (-6.3413, 1.5)
  line L16 (230.642, -112.3) -> (230.642, -113.3)
  line L17 (230.642, -113.3) -> (222.602, -113.3)
  line L18 (-36.12, -117.7958) -> (-31.338, -117.8)
  line L19 (222.602, -113.3) -> (222.602, -112.3)
  line L20 (-28.337, -113.3) -> (-28.337, -112.3)
  line L21 (-29.3375, -113.3) -> (-29.338, -113.3)
  arc A2 (-38.6178, -115.2937) -> (-36.12, -117.7958) centre (-36.1178, -115.2958) ccw
  line L22 (57.336, -112.3) -> (-20.297, -112.3)
  line L23 (8.02, 1) -> (8.02, 0)
  line L24 (-29.3375, -112.3) -> (-29.3375, -113.3)
  line L25 (-33.0995, -112.3) -> (-33.0995, 1.5)
  line L26 (-29.338, -112.3) -> (-33.0995, -112.3)
  line L27 (57.336, -113.3) -> (57.336, -112.3)
  line L28 (-20.297, -113.3) -> (-28.337, -113.3)
  line L29 (-29.338, -113.3) -> (-29.338, -112.3)
  line L30 (-20.297, -112.3) -> (-20.297, -113.3)
  line L31 (301.275, 5.5) -> (-36.0995, 5.5)
  line L32 (-38.5995, -94.25) -> (-38.6178, -115.2937)
  line L33 (298.2751, -76.2) -> (298.2751, -93.25)
  line L34 (298.275, -95.25) -> (298.275, -95.25)
  line L35 (298.275, -76.2) -> (298.275, -76.2)
  line L36 (-6.3413, 1.5) -> (-6.3413, 0)
  line L37 (-38.5995, 3) -> (-38.5995, -94.25)
  arc A3 (303.775, 3) -> (301.275, 5.5) centre (301.275, 3) ccw
  line L38 (298.2751, -74.2) -> (298.275, -74.2)
  line L39 (-28.337, 3) -> (-28.337, 1.5)
  line L40 (-33.0995, 1.5) -> (-28.3375, 1.5)
  line L41 (-0.02, 0) -> (-0.02, 1)
  arc A4 (-36.0995, 5.5) -> (-38.5995, 3) centre (-36.0995, 3) ccw
  line L42 (-31.338, -117.8) -> (302.0217, -117.8)
  line L43 (-6.3413, 0) -> (-0.02, 0)
  line L44 (298.275, -57.15) -> (298.275, -57.15)
  line L45 (-0.02, 1) -> (8.02, 1)
  line L46 (8.02, 0) -> (171.43, 0)
  line L47 (-28.3375, 3) -> (-28.337, 3)
  line L48 (290.235, 0) -> (290.235, 1)
  line L49 (290.235, 1) -> (298.275, 1)
  line L50 (298.2751, -57.15) -> (298.2751, -74.2)
  line L51 (298.275, 1) -> (298.275, -57.15)
  line L52 (222.602, -112.3) -> (65.376, -112.3)
  line L53 (-33.0995, -112.3) -> (-33.0995, 1.5)
  line L54 (301.275, 5.5) -> (-36.0995, 5.5)
  line L55 (-31.338, -117.8) -> (302.0217, -117.8)
  line L56 (57.336, -112.3) -> (-20.297, -112.3)
  line L57 (8.02, 0) -> (171.43, 0)
  line L58 (290.2351, -112.3) -> (230.642, -112.3)
  line L59 (298.2751, -95.25) -> (298.2751, -113.3)
  line L60 (298.275, -76.2) -> (298.275, -76.2)
  line L61 (298.275, -74.2) -> (298.275, -76.2)
  line L62 (298.2751, -76.2) -> (298.2751, -93.25)
  line L63 (298.2751, -93.25) -> (298.275, -93.25)
  line L64 (298.275, -93.25) -> (298.275, -95.25)
  line L65 (290.2351, -113.3) -> (290.2351, -112.3)
  arc A5 (302.0217, -117.8) -> (304.5217, -115.3) centre (302.0374, -115.3157) ccw
  line L66 (179.47, 0) -> (290.235, 0)
  line L67 (298.2751, -113.3) -> (290.2351, -113.3)
  line L68 (304.5217, -115.3) -> (303.775, 3)
  line L69 (298.275, -95.25) -> (298.275, -95.25)
  line L70 (57.336, -113.3) -> (57.336, -112.3)
  line L71 (65.376, -113.3) -> (57.336, -113.3)
  line L72 (-29.338, -113.3) -> (-29.338, -112.3)
  line L73 (-6.3413, 1.5) -> (-6.3413, 0)
  line L74 (-29.3375, -113.3) -> (-29.338, -113.3)
  line L75 (-29.3375, -112.3) -> (-29.3375, -113.3)
  line L76 (-28.3375, 1.5) -> (-28.3375, 3)
  line L77 (-28.337, 1.5) -> (-6.3413, 1.5)
  line L78 (-28.337, -112.3) -> (-29.3375, -112.3)
  line L79 (-28.337, -113.3) -> (-28.337, -112.3)
  line L80 (-28.3375, 3) -> (-28.337, 3)
  line L81 (-20.297, -113.3) -> (-28.337, -113.3)
  line L82 (65.376, -112.3) -> (65.376, -113.3)
  line L83 (-20.297, -112.3) -> (-20.297, -113.3)
  line L84 (-29.338, -112.3) -> (-33.0995, -112.3)
  line L85 (8.02, 1) -> (8.02, 0)
  line L86 (-28.337, 3) -> (-28.337, 1.5)
  arc A6 (-38.6178, -115.2937) -> (-36.12, -117.7958) centre (-36.1178, -115.2958) ccw
  line L87 (-38.5995, -94.25) -> (-38.6178, -115.2937)
  line L88 (-38.5995, 3) -> (-38.5995, -94.25)
  line L89 (-0.02, 0) -> (-0.02, 1)
  line L90 (-33.0995, 1.5) -> (-28.3375, 1.5)
  line L91 (-6.3413, 0) -> (-0.02, 0)
  arc A7 (-36.0995, 5.5) -> (-38.5995, 3) centre (-36.0995, 3) ccw
  line L92 (-0.02, 1) -> (8.02, 1)
  line L93 (-36.12, -117.7958) -> (-31.338, -117.8)
  line L94 (298.275, -93.25) -> (298.275, -95.25)
  line L95 (298.2751, -113.3) -> (290.2351, -113.3)
  line L96 (290.2351, -113.3) -> (290.2351, -112.3)
  line L97 (298.2751, -93.25) -> (298.275, -93.25)
  line L98 (298.275, -74.2) -> (298.275, -76.2)
  line L99 (298.2751, -74.2) -> (298.275, -74.2)
  line L100 (290.235, 0) -> (290.235, 1)
  line L101 (179.47, 1) -> (179.47, 0)
  line L102 (230.642, -113.3) -> (222.602, -113.3)
  line L103 (179.47, 1) -> (179.47, 0)
  line L104 (171.43, 1) -> (179.47, 1)
  line L105 (222.602, -112.3) -> (65.376, -112.3)
  line L106 (65.376, -112.3) -> (65.376, -113.3)
  line L107 (65.376, -113.3) -> (57.336, -113.3)
  line L108 (171.43, 0) -> (171.43, 1)
  line L109 (171.43, 1) -> (179.47, 1)
  dimension "d61" = 5.5
  dimension "d62" = 5.5
  dimension "d63" = 6.2339
  dimension "d64" = 5.5125
  dimension "d65" = 5.5
  dimension "d66" = 6.2276
  dimension "d67" = 5.5188
  constraint coincident L5.start L8.start
  constraint perpendicular L0 L8
  constraint coincident L8.end L59
  constraint coincident L4.end L7.start
  constraint perpendicular L7 L48
  constraint coincident L7.end L51
  measures "d61" distance of L42 L58
  measures "d62" distance of L4 L31
  measures "d63" distance of L0.end L3
  measures "d64" distance of L1.start L3
  measures "d65" distance of L25 L37
  measures "d66" distance of L8.end L3
  measures "d67" distance of L7.end L68
